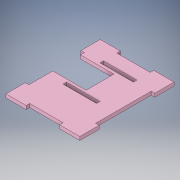
# Autodesk Inventor part: HOMBRO_TAPA.LAT
Saved by Autodesk Inventor 2019 (Build 230136000, 136)
## iProperties
Created: 2020-02-12
Part Number: HOMBRO_TAPA.LAT
Material: Genérico
Document SubType Name: Modeling
Designer: omar-
Density: 1 g/cm^3
Appearance: Valor por defecto
Author: omar-
Autodesk Inventor part; units mm, degrees
ref_plane "YZ Plane" through (0, 0, 0) normal (1, 0, 0) x (0, 1, 0)
ref_plane "XZ Plane" through (0, 0, 0) normal (0, 1, 0) x (-1, 0, 0)
ref_plane "XY Plane" through (0, 0, 0) normal (0, 0, 1) x (1, 0, 0)
sketch "Boceto2" plane through (0, 0, 0) normal (0, 1, 0) x (-1, 0, 0)
  line L0 (33.18, 42.36) -> (-33.18, 42.36)
  line L1 (-33.18, 42.36) -> (-33.18, -42.36)
  line L2 (-33.18, -42.36) -> (33.18, -42.36)
  line L3 (33.18, -42.36) -> (33.18, 42.36)
  line L4 (33.18, 42.36) -> (-33.18, -42.36) construction
  line L5 (-33.18, 42.36) -> (33.18, -42.36) construction
  line L6 (15, 42.36) -> (-15, 42.36)
  line L7 (-15, 42.36) -> (-15, 39.18)
  line L8 (-15, 39.18) -> (15, 39.18)
  line L9 (15, 39.18) -> (15, 42.36)
  line L10 (15, 42.36) -> (-15, 39.18) construction
  line L11 (-15, 42.36) -> (15, 39.18) construction
  line L12 (15, 9.18) -> (-15, 9.18)
  line L13 (-15, 9.18) -> (-15, 6)
  line L14 (-15, 6) -> (15, 6)
  line L15 (15, 6) -> (15, 9.18)
  line L16 (15, 9.18) -> (-15, 6) construction
  line L17 (-15, 9.18) -> (15, 6) construction
  line L18 (15, -24) -> (-15, -24)
  line L19 (-15, -24) -> (-15, -27.18)
  line L20 (-15, -27.18) -> (15, -27.18)
  line L21 (15, -27.18) -> (15, -24)
  line L22 (15, -24) -> (-15, -27.18) construction
  line L23 (-15, -24) -> (15, -27.18) construction
  line L24 (15, -39.18) -> (-15, -39.18)
  line L25 (-15, -39.18) -> (-15, -42.36)
  line L26 (-15, -42.36) -> (15, -42.36)
  line L27 (15, -42.36) -> (15, -39.18)
  line L28 (15, -39.18) -> (-15, -42.36) construction
  line L29 (-15, -39.18) -> (15, -42.36) construction
  line L30 (-30, 25) -> (-33.18, 25)
  line L31 (-33.18, 25) -> (-33.18, -25)
  line L32 (-33.18, -25) -> (-30, -25)
  line L33 (-30, -25) -> (-30, 25)
  line L34 (-30, 25) -> (-33.18, -25) construction
  line L35 (-33.18, 25) -> (-30, -25) construction
  line L36 (33.18, 25) -> (30, 25)
  line L37 (30, 25) -> (30, -25)
  line L38 (30, -25) -> (33.18, -25)
  line L39 (33.18, -25) -> (33.18, 25)
  line L40 (33.18, 25) -> (30, -25) construction
  line L41 (30, 25) -> (33.18, -25) construction
  line L42 (30, 3.5) -> (0, 3.5)
  line L43 (0, 3.5) -> (0, -21.5)
  line L44 (0, -21.5) -> (30, -21.5)
  line L45 (30, -21.5) -> (30, 3.5)
  line L46 (30, 3.5) -> (0, -21.5) construction
  line L47 (0, 3.5) -> (30, -21.5) construction
  point P0 (0, 0)
  point P1 (0, 40.77)
  point P2 (0, 7.59)
  point P3 (0, -25.59)
  point P4 (0, -40.77)
  point P5 (-31.59, 0)
  point P6 (31.59, 0)
  point P7 (15, -9)
  dimension "d37" = 84.72
  dimension "d38" = 66.36
  dimension "d39" = 30
  dimension "d40" = 3.18
  dimension "d41" = 0
  dimension "d42" = 3.18
  dimension "d43" = 30
  dimension "d44" = 30
  dimension "d45" = 3.18
  dimension "d46" = 30
  dimension "d47" = 30
  dimension "d48" = 12
  dimension "d49" = 50
  dimension "d50" = 0
  dimension "d51" = 0
  dimension "d52" = 50
  dimension "d53" = 15
  dimension "d54" = 25
  dimension "d59" = 30
  constraints: 96 end point, 16 midpoint, 16 parallel, 8 horizontal, 8 perpendicular, 7 collinear, 4 equal length
  measures "d37" distance of L1.end L0.end
  measures "d38" distance of L1.end L2.end
  measures "d39" distance of L7.end L8.end
  measures "d40" distance of L8.end L6.start
  measures "d41" horizontal distance of point (0, 40.77) point (0, 0)
  measures "d42" distance of L14.end L12.start
  measures "d43" distance between parallel lines of L8 L12
  measures "d44" distance of L19.end L20.end
  measures "d45" distance of L20.end L18.start
  measures "d46" distance between parallel lines of L18 L14
  measures "d47" distance of L26.end L25.end
  measures "d48" distance between parallel lines of L20 L24
  measures "d49" distance of L32.end L30.start
  measures "d50" vertical distance of point (-31.59, 0) point (0, 0)
  measures "d51" vertical distance of point (0, 0) point (31.59, 0)
  measures "d52" distance of L36.end L37.end
  measures "d53" distance from line of L14 point (15, -9)
  measures "d54" distance of L42.end L43.end
  measures "d59" distance between parallel lines of L43 L37
extrude "Extrusión2" add sketch "Boceto2" along normal blind 3.18 contours L3 L36 L37 L42 L43 L44 L38 L2 L27 L24 L25 L1 L32 L33 L30 L0 L7 L8 L9
